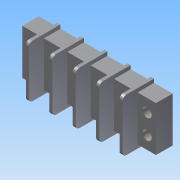
# Autodesk Inventor part: Terminal Block
Saved by Autodesk Inventor 2013 (Build 170138000, 138)
## iProperties
Created: 2012-05-24
Part Number: Terminal Block
Material: Generic
Document SubType Name: Modeling
Designer: dgitz
Density: 1 g/cm^3
Categories: <MemberInstance><Categories><Category DisplayName="" Mnemonic="CABLEANDHARNESS" InternalName="e4a7e005-5e42-4d16-b293-125e7f0d0512"><Category DisplayName="" Mnemonic="CONNECTORS" InternalName="6f634eba-a678-4820-a31d-2c2d5ee6728e"><CategoryParameter DisplayName="" Mnemonic="REFDES" InternalName="c3740e8c-60ab-4d5d-8584-52b73222f2f0"/><Category DisplayName="" Mnemonic="DISCRETEWIRE" InternalName="9a3407de-09b2-4cdb-8c40-9708d5144a28"/></Category></Category></Categories><FamilyTemplate><FamilyTemplateParameters></FamilyTemplateParameters></FamilyTemplate><CategoryParameterMap><ParamToTemplateMap><ParamToTemplate CategoryParameter="//CategoryParameter[@InternalName='c3740e8c-60ab-4d5d-8584-52b73222f2f0']" ConstantValue="U?"/></ParamToTemplateMap></CategoryParameterMap></MemberInstance>
GlobalPropertyList: <PropertyList/>
Author: dgitz
Autodesk Inventor part; units mm, degrees
ref_plane "YZ Plane" through (0, 0, 0) normal (1, 0, 0) x (0, 1, 0)
ref_plane "XZ Plane" through (0, 0, 0) normal (0, 1, 0) x (-1, 0, 0)
sketch "Sketch1" plane through (0, 0, 0) normal (0, 0, 1) x (1, 0, 0)
  line L0 (-27.559, 9.271) -> (27.559, 9.271)
  line L1 (27.559, 9.271) -> (27.559, -9.271)
  line L2 (27.559, -9.271) -> (-27.559, -9.271)
  line L3 (-27.559, -9.271) -> (-27.559, 9.271)
  line L4 (-27.559, 9.271) -> (27.559, -9.271) construction
  point P0 (0, 0)
  point P1 (0, 0)
  dimension "d0" = 55.118
  dimension "d1" = 18.542
  constraints: 10 end point, 2 parallel, 1 coincident, 1 horizontal, 1 midpoint, 1 perpendicular
  measures "d0" distance of L0.start L0.end
  measures "d1" distance of L2.end L0.start
extrude "Extrusion1" add sketch "Sketch1" along normal blind 6.858
sketch "Sketch2" plane through (0, 0, 6.858) normal (0, 0, 1) x (1, 0, 0)
  line L0 (27.559, -9.271) -> (-27.559, -9.271) projected
  circle A0 centre (-23.876, 4.064) radius 1.905
  circle A1 centre (-23.876, -4.064) radius 1.905
  circle A2 centre (23.876, 4.064) radius 1.905
  circle A3 centre (23.876, -4.064) radius 1.905
  line L1 (-23.876, 4.064) -> (-23.876, -4.064) construction
  line L2 (-23.876, -4.064) -> (23.876, -4.064) construction
  line L3 (23.876, -4.064) -> (23.876, 4.064) construction
  line L4 (23.876, 4.064) -> (-23.876, 4.064) construction
  line L5 (-23.876, 4.064) -> (23.876, -4.064) construction
  point P0 (0, 0)
  point P1 (0, 0)
  dimension "d4" = 3.81
  dimension "d5" = 4.318
  dimension "d6" = 43.942
  constraints: 10 end point, 4 centre point, 3 equal radius, 2 vertical, 1 coincident, 1 horizontal, 1 midpoint, 1 parallel
  measures "d4" diameter of A0
extrude "Extrusion2" cut sketch "Sketch2" against normal up to surface (6.858 mm away)
ref_plane "Work Plane1" through (19.939, -9.271, 0) normal (1, 0, 0) x (0, 0, -1)
sketch "Sketch3" plane through (19.939, -9.271, 0) normal (1, 0, 0) x (0, 0, -1)
  line L0 (0, 20.066) -> (-11.4173, 20.066)
  line L1 (-13.0048, 18.4785) -> (-13.0048, 0.0635)
  line L2 (-11.4173, -1.524) -> (0, -1.524)
  line L3 (0, -1.524) -> (0, 0)
  line L4 (0, 0) -> (-6.858, 0)
  line L5 (-6.858, 0) -> (-6.858, 18.542)
  line L6 (-6.858, 18.542) -> (0, 18.542)
  line L7 (0, 18.542) -> (0, 20.066)
  line L8 (0, 18.542) -> (0, 0) projected
  line L9 (-6.858, 18.542) -> (-6.858, 0) projected
  arc A0 (-11.4173, 20.066) -> (-13.0048, 18.4785) centre (-11.4173, 18.4785) ccw
  arc A1 (-13.0048, 0.0635) -> (-11.4173, -1.524) centre (-11.4173, 0.0635) ccw
  point P0 (0, 9.271)
  dimension "d10" = 1.524
  dimension "d11" = 13.0048
  dimension "d12" = 1.5875
  constraints: 16 end point, 6 parallel, 4 point on circle, 4 tangent, 2 centre point, 1 collinear, 1 equal radius, 1 horizontal, 1 perpendicular, 1 point on line
  measures "d10" distance of L6.end L0.start
  measures "d11" distance between parallel lines of L8 L1
  measures "d12" radius of A0
extrude "Extrusion3" add sketch "Sketch3" against normal blind 1.27 contours L7 L6 L5 L4 L3 L2 A1 L1 A0 L0
pattern_linear "Rectangular Pattern1" count 5 spacing 9.652 along (-1, 0, 0) of "Extrusion3"
sketch "Sketch4" plane through (0, 0, 6.858) normal (0, 0, 1) x (1, 0, 0)
  line L0 (-18.669, 9.2075) -> (-18.669, -9.2075) projected
  line L1 (-10.287, 9.2075) -> (-10.287, -9.2075) projected
  line L2 (-9.017, 9.2075) -> (-9.017, -9.2075) projected
  line L3 (-0.635, 9.2075) -> (-0.635, -9.2075) projected
  line L4 (0.635, 9.2075) -> (0.635, -9.2075) projected
  line L5 (9.017, 9.2075) -> (9.017, -9.2075) projected
  line L6 (10.287, 9.2075) -> (10.287, -9.2075) projected
  line L7 (18.669, 9.2075) -> (18.669, -9.2075) projected
  line L8 (19.939, 9.2075) -> (19.939, -9.2075) projected
  circle A0 centre (-14.478, 4.064) radius 1.397
  circle A1 centre (-14.478, -4.064) radius 1.397
  line L9 (-14.478, 4.064) -> (-14.478, -4.064) construction
  line L10 (-37.6243, 0) -> (37.6243, 0) construction
  circle A2 centre (-4.826, 4.064) radius 1.397
  circle A3 centre (-4.826, -4.064) radius 1.397
  circle A4 centre (4.826, 4.064) radius 1.397
  circle A5 centre (4.826, -4.064) radius 1.397
  circle A6 centre (14.478, 4.064) radius 1.397
  circle A7 centre (14.478, -4.064) radius 1.397
  point P0 (0, 0)
  point P1 (0, 0)
  point P2 (-14.478, 0)
  dimension "d18" = 2.794
  dimension "d19" = 5.334
  dimension "d21" = 4.191
  dimension "d28" = 9.652
  constraints: 8 centre point, 4 end point, 2 horizontal, 2 midpoint, 1 coincident, 1 equal radius, 1 point on line, 1 vertical, 12 other
  measures "d18" diameter of A0
  measures "d21" distance from line of L9.start L0
  measures "d28" distance of L9.start A2.centre
extrude "Extrusion4" cut sketch "Sketch4" against normal blind 3.175
sketch "Sketch5" plane through (0, 0, 6.858) normal (0, 0, 1) x (1, 0, 0)
  circle A0 centre (-14.478, -4.064) radius 1.397 projected
sketch "Sketch6" plane through (0, 0, 6.858) normal (0, 0, 1) x (1, 0, 0)
  circle A0 centre (-14.478, 4.064) radius 1.397 projected
sketch "Sketch7" plane through (0, 0, 6.858) normal (0, 0, 1) x (1, 0, 0)
  circle A0 centre (-4.826, -4.064) radius 1.397 projected
sketch "Sketch8" plane through (0, 0, 6.858) normal (0, 0, 1) x (1, 0, 0)
  circle A0 centre (-4.826, 4.064) radius 1.397 projected
sketch "Sketch9" plane through (0, 0, 6.858) normal (0, 0, 1) x (1, 0, 0)
  circle A0 centre (4.826, 4.064) radius 1.397 projected
sketch "Sketch10" plane through (0, 0, 6.858) normal (0, 0, 1) x (1, 0, 0)
  circle A0 centre (14.478, -4.064) radius 1.397 projected
sketch "Sketch11" plane through (0, 0, 6.858) normal (0, 0, 1) x (1, 0, 0)
  circle A0 centre (23.876, 4.064) radius 1.905 projected
sketch "Sketch12" plane through (0, 0, 6.858) normal (0, 0, 1) x (1, 0, 0)
  circle A0 centre (23.876, -4.064) radius 1.905 projected
body "Solid1"
